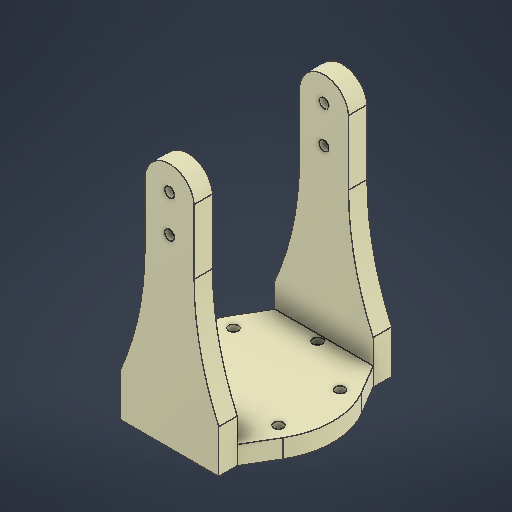
# Autodesk Inventor part: MOUNTING-COUPLE
Saved by Autodesk Inventor 2025.3 (Build 293356030, 356C)
## iProperties
Created: 2025-08-29
Part Number: MOUNTING-COUPLE
Material: Generic
Document SubType Name: Modeling
Designer: lstk1ng
Density: 1 g/cm^3
Appearance: Default
Author: lstk1ng
Autodesk Inventor part; units mm, degrees
ref_plane "YZ Plane" through (0, 0, 0) normal (1, 0, 0) x (0, 1, 0)
ref_plane "XZ Plane" through (0, 0, 0) normal (0, 1, 0) x (-1, 0, 0)
ref_plane "XY Plane" through (0, 0, 0) normal (0, 0, 1) x (1, 0, 0)
sketch "Sketch1" plane through (0, 0, 0) normal (0, 1, 0) x (-1, 0, 0)
  circle A0 centre (0, 0) radius 50 construction
  circle A1 centre (50, 0) radius 4
  line L0 (0, 0) -> (43.3013, -25) construction
  line L1 (0, 0) -> (50, 0) construction
  circle A2 centre (43.3013, -25) radius 4
  circle A3 centre (43.3013, 25) radius 4
  circle A4 centre (0, 50) radius 4
  circle A5 centre (-43.3013, 25) radius 4
  circle A6 centre (-43.3013, -25) radius 4
  circle A7 centre (0, -50) radius 4
  line L2 (25, 55.25) -> (-25, 55.25)
  arc A8 (-53.8355, 31.903) -> (-62.5784, 0) centre (0, 0) ccw
  arc A9 (62.5784, 0) -> (53.8355, 31.903) centre (0, 0) ccw
  line L3 (0, 55.25) -> (40, 55.25)
  line L4 (0, 55.25) -> (-40, 55.25)
  line L5 (40, 55.25) -> (53.8355, 31.903)
  line L6 (-40, 55.25) -> (-53.8355, 31.903)
  line L7 (62.5784, 0) -> (-62.5784, 0) construction
  arc A10 (-62.5784, 0) -> (-53.8355, -31.903) centre (0, 0) ccw
  arc A11 (53.8355, -31.903) -> (62.5784, 0) centre (0, 0) ccw
  line L8 (0, -55.25) -> (40, -55.25)
  line L9 (0, -55.25) -> (-40, -55.25)
  line L10 (40, -55.25) -> (53.8355, -31.903)
  line L11 (-40, -55.25) -> (-53.8355, -31.903)
  point P0 (-25, 55.25)
  dimension "d1" = 100
  dimension "d2" = 8
  dimension "d3" = 30
  dimension "d4" = 8
  dimension "d7" = 360
  dimension "d35" = 40
  dimension "d36" = 40
  dimension "d49" = 110.5
  constraints: 24 end point, 12 centre point, 10 point on circle, 5 symmetric about line, 3 coincident, 3 horizontal, 3 point on line, 2 tangent, 1 equal length, 1 midpoint, 15 other
  measures "d1" diameter of A0
  measures "d2" diameter of A1
  measures "d3" angle of L0 L1
  measures "d4" diameter of A2
  measures "d35" distance of L3.start L3.end
  measures "d36" distance of L3.start L4.end
  measures "d49" distance between parallel lines of L8 L3
extrude "Extrusion1" add sketch "Sketch1" along normal blind 15
sketch "Sketch4" plane through (-40, 0, 55.25) normal (0, 0, 1) x (1, 0, 0)
  line L0 (40, 200) -> (40, 184) construction
  line L1 (40, 184) -> (40, 180) construction
  circle A0 centre (40, 180) radius 4
  line L2 (40, 180) -> (40, 150) construction
  circle A1 centre (40, 150) radius 4
  arc A2 (59.9595, 181.2724) -> (20.0405, 181.2724) centre (40, 180) ccw
  line L3 (0, 0) -> (0, 15) projected
  line L4 (0, 15) -> (0, 0)
  line L5 (80, 0) -> (80, 15) projected
  line L6 (0, 0) -> (80, 0)
  line L7 (80, 0) -> (80, 15)
  line L8 (40, 0) -> (40, 15) construction
  line L9 (40, 146) -> (40, 200) construction
  line L10 (20.0405, 181.2724) -> (20.0405, 131.2724)
  line L11 (0, 15) -> (0, 35)
  line L12 (59.9595, 181.2724) -> (59.9595, 128.6983)
  line L13 (0, 15) -> (80, 15) projected
  line L14 (80, 15) -> (80, 35)
  arc A3 (0, 35) -> (20.0405, 131.2724) centre (-221.2208, 131.2724) ccw
  arc A4 (59.9595, 128.6983) -> (80, 35) centre (289.0202, 128.6983) ccw
  dimension "d42" = 8
  dimension "d37" = 200
  dimension "d38" = 16
  dimension "d39" = 4
  dimension "d40" = 8
  dimension "d41" = 30
  dimension "d50" = 50
  dimension "d51" = 20
  dimension "d52" = 20
  constraints: 24 end point, 7 point on circle, 6 vertical, 4 centre point, 3 coincident, 3 point on line, 2 perpendicular, 2 tangent, 1 collinear, 1 vertical alignment, 2 other
  measures "d37" distance of L8.start L0.start
  measures "d38" distance of L0.start L0.end
  measures "d39" distance of L0.end L1.end
  measures "d40" diameter of A0
  measures "d41" distance of L2.start L2.end
  measures "d50" distance of L10.start L10.end
  measures "d51" distance of L3.end L11.end
  measures "d52" distance of L5.end L14.end
extrude "Extrusion3" add sketch "Sketch4" along normal blind 15
mirror "Mirror2" about plane through (0, 0, 0) normal (0, 0, 1) of "Extrusion3"
body "Solid1"
